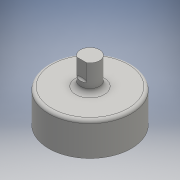
# Autodesk Inventor part: sprag_fill
Saved by Autodesk Inventor 2016 (Build 200138000, 138)
## iProperties
Created: 2017-07-02
Part Number: sprag_fill
Material: Generic
Document SubType Name: Modeling
Designer: ALIREZA
Density: 1 g/cm^3
Appearance: Default
Author: ALIREZA
Autodesk Inventor part; units mm, degrees
ref_plane "YZ Plane" through (0, 0, 0) normal (1, 0, 0) x (0, 1, 0)
ref_plane "XZ Plane" through (0, 0, 0) normal (0, 1, 0) x (-1, 0, 0)
ref_plane "XY Plane" through (0, 0, 0) normal (0, 0, 1) x (1, 0, 0)
sketch "Sketch1" plane through (0, 0, 0) normal (0, 0, 1) x (1, 0, 0)
  circle A0 centre (0, 0) radius 11
  dimension "d0" = 22
  constraints: 1 centre point, 1 coincident
  measures "d0" diameter of A0
sketch "Sketch2" plane through (0, 0, 0) normal (0, 0, 1) x (1, 0, 0)
  circle A0 centre (0, 0) radius 13
  dimension "d1" = 26
  constraints: 1 centre point, 1 coincident
  measures "d1" diameter of A0
extrude "Extrusion1" add sketch "Sketch2" along normal blind 10.5
extrude "Extrusion2" cut sketch "Sketch1" along normal blind 9
fillet "Fillet1" radius 0.5 1 edges at (-11, 0, 9)
sketch "Sketch3" plane through (0, 0, 10.5) normal (0, 0, 1) x (1, 0, 0)
  circle A0 centre (0, 0) radius 3
  dimension "d7" = 6
  constraints: 1 centre point, 1 coincident
  measures "d7" diameter of A0
extrude "Extrusion3" add sketch "Sketch3" along normal blind 8.5
fillet "Fillet2" radius 1 1 edges at (-13, 0, 10.5)
fillet "Fillet3" radius 1.5 1 edges at (-3, 0, 10.5)
sketch "Sketch4" plane through (0, 0, 19) normal (0, 0, 1) x (1, 0, 0)
  arc A0 (-1.5, -2.5981) -> (1.5154, -2.5891) centre (0, 0) ccw
  line L0 (-1.5, -2.5981) -> (1.5154, -2.5891)
  circle A1 centre (0, 0) radius 3 projected
  constraints: 2 end point, 2 point on circle, 1 centre point, 2 other
extrude "Extrusion4" cut sketch "Sketch4" against normal blind 5.5 contours L0 A0
sketch "Sketch5" plane through (0, 0, 10.5) normal (0, 0, 1) x (1, 0, 0)
  point P0 (0, 0)
sketch "Sketch8" plane through (0, 0, 0) normal (0, 0, -1) x (-1, 0, 0)
  circle A0 centre (0, 0) radius 11 projected
  line L0 (0.1347, -8.9459) -> (-0.865, -8.9703)
  line L1 (-0.865, -8.9703) -> (-0.8163, -10.9697)
  line L2 (0.1347, -8.9459) -> (1.1347, -8.9459)
  line L3 (1.1347, -8.9459) -> (1.1347, -10.9413)
  dimension "d27" = 1
  dimension "d28" = 1
  dimension "d32" = 2
  constraints: 8 end point, 2 perpendicular, 2 point on circle, 1 horizontal
  measures "d27" distance of L0.start L0.end
  measures "d28" distance of L0.start L2.end
  measures "d32" distance of L0.end L1.end
extrude "Extrusion7" add sketch "Sketch8" against normal up to next contours L1 L0 L2 L3 A0 picked at (-0.2987, -9.6383)
fillet "Fillet4" radius 1 1 edges at (0.0077, -2.5936, 13.5)
sketch "Sketch9" plane through (0, 0, 0) normal (0, 0, -1) x (-1, 0, 0)
  line L0 (0.1347, -8.9459) -> (1.1347, -8.9459) projected
  line L1 (-0.9467, -11.1508) -> (0.6347, -11.1508)
  line L2 (0.6347, -11.1508) -> (0.6347, -8.9459)
  line L3 (0.6347, -8.9459) -> (-0.9467, -8.9459)
  line L4 (-0.9467, -8.9459) -> (-0.9467, -11.1508)
  point P0 (0, 0)
  constraints: 8 end point, 2 parallel, 1 horizontal, 1 midpoint, 1 perpendicular
extrude "Extrusion8" add sketch "Sketch9" against normal up to surface (9 mm away)
sketch "Sketch10" plane through (0, 0, 0) normal (0, 0, -1) x (-1, 0, 0)
  line L0 (-2.2069, -6.8091) -> (2.0454, -6.8091)
  line L1 (2.0454, -6.8091) -> (2.0454, -9.1774)
  line L2 (2.0454, -9.1774) -> (-2.2069, -9.1774)
  line L3 (-2.2069, -9.1774) -> (-2.2069, -6.8091)
  point P0 (0, 0)
  constraints: 8 end point, 2 parallel, 1 horizontal, 1 perpendicular
extrude "Extrusion9" cut sketch "Sketch10" against normal up to surface (9 mm away)
body "Solid1"
